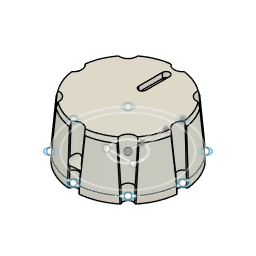
CHORDS Knob 2 (Autodesk Fusion 360 design; units mm, degrees)
Autodesk Fusion 360 part; units mm, degrees
sketch "Sketch1" plane through (0, 0, 0) normal (0, 1, 0) x (1, 0, 0)
  circle A0 centre (0, 0) radius 3
  line L0 (0, 0) -> (0, 3) construction
  line L1 (0, 3) -> (0, -1.6) construction
  line L2 (0, -1.6) -> (-2.5377, -1.6)
  line L3 (0, -1.6) -> (2.5377, -1.6)
  circle A1 centre (0, 0) radius 3.17
  line L4 (0, -1.72) -> (2.5377, -1.72)
  line L5 (0, -1.72) -> (-2.5377, -1.72)
  circle A2 centre (0, 0) radius 10
  circle A3 centre (0, 0) radius 11.5
  line L6 (0, 11.5) -> (0, 10) construction
  circle A4 centre (0, 11.5) radius 1
  circle A5 centre (-8.1317, 8.1317) radius 1
  circle A6 centre (-11.5, 0) radius 1
  circle A7 centre (-8.1317, -8.1317) radius 1
  circle A8 centre (0, -11.5) radius 1
  circle A9 centre (8.1317, -8.1317) radius 1
  circle A10 centre (11.5, 0) radius 1
  line L7 (2.5377, -1.72) -> (2.9, -1.72)
  line L8 (-2.5377, -1.72) -> (-2.8, -1.72)
  circle A11 centre (8.1317, 8.1317) radius 1
  line L9 (0, 0) -> (0, 8) construction
  line L10 (-0.75, 8) -> (-0.75, 3)
  arc A12 (-0.75, 3) -> (0.75, 3) centre (0, 3) ccw
  line L11 (0.75, 3) -> (0.75, 8)
  arc A13 (0.75, 8) -> (-0.75, 8) centre (0, 8) ccw
  line L12 (0, 8) -> (0, 3) construction
  dimension "d1" = 6
  dimension "d3" = 4.6
  dimension "d4" = 0.17
  dimension "d5" = 0.12
  dimension "d6" = 20
  dimension "d7" = 1.5
  dimension "d10" = 2
  dimension "d12" = 360
  dimension "d62" = 8
  dimension "d63" = 5
  dimension "d64" = 1.5
  constraint coincident A0.centre L0.start
  constraint coincident A0 L0.end
  constraint vertical L0
  constraint parallel L0 L1
  constraint coincident A0 L2.end
  constraint perpendicular L1 L2
  constraint coincident A0 L3.end
  constraint perpendicular L1 L3
  constraint concentric A0 A2
  constraint coincident A3 L6.start
  constraint coincident A2 L6.end
  constraint vertical L6
  constraint coincident L6.start A4.centre
  constraint parallel L4 L7
  constraint parallel L5 L8
  constraint parallel L1 L9
  constraint tangent L10 A12
  constraint tangent A12 L11
  constraint parallel L10 L11
  constraint tangent L11 A13
  constraint tangent L10 A13
  constraint coincident L9 L0.end
  constraint coincident L9.end A13.centre
  measures "d1" diameter of A0
  measures "d3" distance of L0.end L1.end
  measures "d6" diameter of A2
  measures "d10" diameter of A4
  measures "d62" distance of A0.centre L9.end
  measures "d63" distance of L9.end L0.end
  measures "d64" diameter of A12
extrude "Extrude1" add sketch "Sketch1" along normal blind 10 draft -4.5 contours A0 L2 L3 A12 | A0 A1 L4 L7 A12 L11 | A0 L2 L3 L4 L5 | A0 A1 L4 L5 L7 L8 | A0 L4 L5 | A0 A12 | A0 A1 L10 A12 L11 | A0 A1 L5 L8 L10 A12 | A1 L10 L11 A13 | A2 | A3 A4 A5 A6 A7 A8 A9 A10 A11
sketch "Sketch2" plane through (0, 0, 0) normal (0, 0, 1) x (1, 0, 0)
  line L0 (0, 0) -> (0, 3.2) construction
  circle A0 centre (0, 3.2) radius 1.4
  dimension "d21" = 2.8
  constraint coincident L0.start origin
  constraint vertical L0
  constraint coincident L0.end A0.centre
  measures "d21" diameter of A0
extrude "Extrude5" cut sketch "Sketch1" along normal blind 8 contours A0 L2 L3 A12 | A0 A1 L4 L7 A12 L11 | A0 L2 L3 L4 L5 | A0 A12 | A0 A1 L10 A12 L11 | A0 A1 L5 L8 L10 A12
chamfer "Chamfer2" distance 1 distance2 0.2 8 edges at (9.8975, 10, 4.0997) (4.0997, 10, 9.8975) (-4.0997, 10, 9.8975) (-9.8975, 10, 4.0997) (-9.8975, 10, -4.0997) (-4.0997, 10, -9.8975) (4.0997, 10, -9.8975) (9.8975, 10, -4.0997) measured on face at (10.5492, 2.2222, 4.1198) measured on face at (4.5463, 2.2222, 10.3725) measured on face at (-4.5463, 2.2222, 10.3725) measured on face at (-10.3725, 2.2222, 4.5463) measured on face at (-10.3725, 2.2222, -4.5463) measured on face at (-4.1198, 2.2222, -10.5492) measured on face at (4.5463, 2.2222, -10.3725) measured on face at (10.3725, 2.2222, -4.5463)
extrude "Extrude7" cut sketch "Sketch1" against normal blind 1.5 from surface at 10 contours A0 A12 | A0 A1 L10 A12 L11 | A1 L10 L11 A13
chamfer "Chamfer4" distance 0.4 distance2 0.75 4 edges at (-0.75, 8.5, -5.5) (0, 8.5, -8.75) (0.75, 8.5, -5.5) (0, 8.5, -2.25) measured on face at (-0.75, 9.5, -6.3333) measured on face at (-0.64, 9.5, -8.3911) measured on face at (0.75, 9.5, -4.6667) measured on face at (-0.6911, 9, -2.7087)
extrude "Extrude8" cut sketch "Sketch2" along normal blind 20
extrude "Extrude9" cut sketch "Sketch1" along normal blind 1 contours A0 A1 L4 L5 L7 L8 | A0 L4 L5
chamfer "Chamfer5" distance 0.4 distance2 1 1 edges at (-2.9555, 0, 1.1463) measured on face at (-1.8207, 0, 8.1405)
fillet "Fillet7" radius 1 2 edges at (2.6628, 4.5, 1.72) (-2.6628, 4.5, 1.72)
extrude "Extrude10" add 1 faces at (4.5327, 0, -7.1615) along direction (0, -1, 0) blind 1.5
fillet "Fillet8" radius 40 8 edges at (0, 0, 10.5) (-7.4246, 0, 7.4246) (-10.5, 0, 0) (-7.4246, 0, -7.4246) (0, 0, -10.5) (7.4246, 0, -7.4246) (10.5, 0, 0) (7.4246, 0, 7.4246)
fillet "Fillet3" radius 0.2 50 edges at (6.8459, 5.2574, 8.72) (7.301, 0.7833, 8.8052) (1.3831, 6.4065, 10.9085) (1.1369, 1.993, 11.286) (1.0636, 0.7833, 11.3888) (-1.3832, 6.4104, 10.9081) (-1.1369, 1.9932, 11.286) (-1.0636, 0.7833, 11.3888) (-6.847, 5.2477, 8.7201) (-7.301, 0.7833, 8.8052) (-8.72, 5.2574, 6.8459) (-8.8052, 0.7833, 7.301) (-11.0076, 5.2477, 1.3245) (-11.3888, 0.7833, 1.0636) (-11.0068, 5.2574, -1.3252) (-11.3888, 0.7833, -1.0636) (-8.7201, 5.2477, -6.847) (-8.8052, 0.7833, -7.301) (-6.8459, 5.2574, -8.72) (-7.301, 0.7833, -8.8052) (-1.3245, 5.2477, -11.0076) (-1.0636, 0.7833, -11.3888) (1.3252, 5.2574, -11.0068) (1.0636, 0.7833, -11.3888) (6.847, 5.2477, -8.7201) (7.301, 0.7833, -8.8052) (8.72, 5.2574, -6.8459) (8.8052, 0.7833, -7.301) (11.0076, 5.2477, -1.3245) (11.3888, 0.7833, -1.0636) (11.0068, 5.2574, 1.3252) (11.3888, 0.7833, 1.0636) (8.7201, 5.2477, 6.847) (8.8052, 0.7833, 7.301) (7.3881, -0.7499, 8.8128) (1.0074, -0.7499, 11.4558) (-1.0074, -0.7499, 11.4558) (-7.3881, -0.7499, 8.8128) (-8.8128, -0.7499, 7.3881) (-11.4558, -0.7499, 1.0074) (-11.4558, -0.7499, -1.0074) (-8.8128, -0.7499, -7.3881) (-7.3881, -0.7499, -8.8128) (1.0074, -0.7499, -11.4558) (-1.0074, -0.7499, -11.4558) (7.3881, -0.7499, -8.8128) (8.8128, -0.7499, -7.3881) (8.8128, -0.7499, 7.3881) (11.4558, -0.7499, 1.0074) (11.4558, -0.7499, -1.0074)
